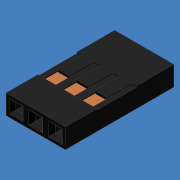
# Autodesk Inventor part: PMW_Terminal
Saved by Autodesk Inventor 2012 (Build 160160000, 160)
## iProperties
Company: Team 801
Created: 2006-06-02
Part Number: PMW_Terminal
Document SubType Name: Modeling
Designer: Jeffrey M
Catalog Web Link: www.team801.org
Density: 1 g/cm^3
Material: Default
Author: Jeffrey M
Autodesk Inventor part; units mm, degrees
ref_plane "YZ Plane" through (0, 0, 0) normal (1, 0, 0) x (0, 1, 0)
ref_plane "XZ Plane" through (0, 0, 0) normal (0, 1, 0) x (-1, 0, 0)
ref_plane "XY Plane" through (0, 0, 0) normal (0, 0, 1) x (1, 0, 0)
sketch "Sketch1" plane through (0, 0, 0) normal (0, 0, 1) x (1, 0, 0)
  line L0 (-23.5871, -5.7068) -> (-15.9671, -5.7068)
  line L1 (-15.9671, -5.7068) -> (-15.9671, -8.2468)
  line L2 (-15.9671, -8.2468) -> (-23.5871, -8.2468)
  line L3 (-23.5871, -8.2468) -> (-23.5871, -5.7068)
  dimension "d0" = 2.54
  dimension "d1" = 7.62
  constraints: 8 end point, 2 parallel, 1 horizontal, 1 perpendicular
  measures "d0" distance of L2.end L0.start
  measures "d1" distance of L0.start L0.end
extrude "Extrusion1" add sketch "Sketch1" along normal blind 13.97
sketch "Sketch2" plane through (0, 0, 13.97) normal (0, 0, 1) x (1, 0, 0)
  line L0 (-23.5871, -5.7068) -> (-15.9671, -5.7068) projected
  line L1 (-23.5871, -8.2468) -> (-23.5871, -5.7068) projected
  line L2 (-15.9671, -8.2468) -> (-23.5871, -8.2468) projected
  line L3 (-23.2061, -6.0878) -> (-21.4281, -6.0878)
  line L4 (-21.4281, -6.0878) -> (-21.4281, -7.8658)
  line L5 (-21.4281, -7.8658) -> (-23.2061, -7.8658)
  line L6 (-23.2061, -7.8658) -> (-23.2061, -6.0878)
  line L7 (-19.7771, -5.7068) -> (-19.7771, -5.9181)
  line L8 (-16.3481, -6.0878) -> (-18.1261, -6.0878)
  line L9 (-18.1261, -6.0878) -> (-18.1261, -7.8658)
  line L10 (-18.1261, -7.8658) -> (-16.3481, -7.8658)
  line L11 (-16.3481, -7.8658) -> (-16.3481, -6.0878)
  line L12 (-20.6661, -6.0878) -> (-18.8881, -6.0878)
  line L13 (-18.8881, -6.0878) -> (-18.8881, -7.8658)
  line L14 (-18.8881, -7.8658) -> (-20.6661, -7.8658)
  line L15 (-20.6661, -7.8658) -> (-20.6661, -6.0878)
  dimension "d4" = 0.381
  dimension "d5" = 0.381
  dimension "d6" = 0.381
  dimension "d7" = 1.778
  dimension "d8" = 1.778
  dimension "d9" = 1.778
  dimension "d10" = 0.762
  dimension "d11" = 0.762
  constraints: 26 end point, 5 parallel, 4 symmetric about line, 2 horizontal, 2 perpendicular, 1 midpoint
  measures "d4" distance between parallel lines of L1 L6
  measures "d5" distance between parallel lines of L0 L3
  measures "d6" distance between parallel lines of L2 L5
  measures "d7" distance of L3.start L3.end
  measures "d8" distance of L12.start L12.end
  measures "d9" distance of L12.end L13.end
  measures "d10" distance between parallel lines of L15 L4
  measures "d11" distance between parallel lines of L9 L13
extrude "Extrusion2" cut sketch "Sketch2" against normal blind 0.381 draft -50
sketch "Sketch3" plane through (0, 0, 13.589) normal (0, 0, 1) x (1, 0, 0)
  line L0 (-22.752, -6.5419) -> (-22.752, -7.4118) projected
  line L1 (-22.752, -7.4118) -> (-21.8821, -7.4118) projected
  line L2 (-21.8821, -7.4118) -> (-21.8821, -6.5419) projected
  line L3 (-21.8821, -6.5419) -> (-22.752, -6.5419) projected
  line L4 (-20.212, -6.5419) -> (-20.212, -7.4118) projected
  line L5 (-20.212, -7.4118) -> (-19.3421, -7.4118) projected
  line L6 (-19.3421, -7.4118) -> (-19.3421, -6.5419) projected
  line L7 (-19.3421, -6.5419) -> (-20.212, -6.5419) projected
  line L8 (-17.672, -6.5419) -> (-17.672, -7.4118) projected
  line L9 (-17.672, -7.4118) -> (-16.8021, -7.4118) projected
  line L10 (-16.8021, -7.4118) -> (-16.8021, -6.5419) projected
  line L11 (-16.8021, -6.5419) -> (-17.672, -6.5419) projected
extrude "Extrusion3" cut sketch "Sketch3" against normal through all
sketch "Sketch4" plane through (0, 0, 0) normal (0, 0, -1) x (-1, 0, 0)
  line L0 (20.212, -7.4118) -> (19.3421, -7.4118) projected
  line L1 (19.3421, -7.4118) -> (19.3421, -6.5419) projected
  line L2 (19.3421, -6.5419) -> (20.212, -6.5419) projected
  line L3 (20.212, -6.5419) -> (20.212, -7.4118) projected
  line L4 (22.752, -7.4118) -> (21.8821, -7.4118) projected
  line L5 (21.8821, -7.4118) -> (21.8821, -6.5419) projected
  line L6 (21.8821, -6.5419) -> (22.752, -6.5419) projected
  line L7 (22.752, -6.5419) -> (22.752, -7.4118) projected
  line L8 (17.672, -7.4118) -> (16.8021, -7.4118) projected
  line L9 (16.8021, -7.4118) -> (16.8021, -6.5419) projected
  line L10 (16.8021, -6.5419) -> (17.672, -6.5419) projected
  line L11 (17.672, -6.5419) -> (17.672, -7.4118) projected
  line L12 (23.2696, -6.0243) -> (21.3646, -6.0243)
  line L13 (21.3646, -6.0243) -> (21.3646, -7.9293)
  line L14 (21.3646, -7.9293) -> (23.2696, -7.9293)
  line L15 (23.2696, -7.9293) -> (23.2696, -6.0243)
  line L16 (18.1896, -6.0243) -> (16.2846, -6.0243)
  line L17 (16.2846, -6.0243) -> (16.2846, -7.9293)
  line L18 (16.2846, -7.9293) -> (18.1896, -7.9293)
  line L19 (18.1896, -7.9293) -> (18.1896, -6.0243)
  line L20 (20.7296, -6.0243) -> (18.8246, -6.0243)
  line L21 (18.8246, -6.0243) -> (18.8246, -7.9293)
  line L22 (18.8246, -7.9293) -> (20.7296, -7.9293)
  line L23 (20.7296, -7.9293) -> (20.7296, -6.0243)
  dimension "d16" = 1.905
  constraints: 24 end point, 2 collinear, 9 other
  measures "d16" distance of L14.end L12.start
extrude "Extrusion4" cut sketch "Sketch4" against normal blind 3.175
sketch "Sketch5" plane through (-23.5871, -5.7068, 0) normal (0, 1, 0) x (1, 0, 0)
  line L0 (7.62, 0) -> (7.62, -13.97) projected
  line L1 (0, 0) -> (0, -13.97) projected
  line L2 (0, -4.826) -> (7.62, -4.826)
  line L3 (7.62, -4.826) -> (7.62, -9.906)
  line L4 (7.62, -9.906) -> (0, -9.906)
  line L5 (0, -9.906) -> (0, -4.826)
  line L6 (0.635, -9.906) -> (2.159, -9.906)
  line L7 (2.159, -9.906) -> (2.159, -8.001)
  line L8 (2.159, -8.001) -> (0.635, -8.001)
  line L9 (0.635, -8.001) -> (0.635, -9.906)
  line L10 (3.81, -9.906) -> (5.334, -9.906)
  line L11 (5.461, -9.906) -> (6.985, -9.906)
  line L12 (6.985, -9.906) -> (6.985, -8.001)
  line L13 (6.985, -8.001) -> (5.461, -8.001)
  line L14 (5.461, -8.001) -> (5.461, -9.906)
  line L15 (3.048, -9.906) -> (4.572, -9.906)
  line L16 (4.572, -9.906) -> (4.572, -8.001)
  line L17 (4.572, -8.001) -> (3.048, -8.001)
  line L18 (3.048, -8.001) -> (3.048, -9.906)
  line L19 (0.635, -8.001) -> (2.159, -8.001)
  line L20 (2.159, -8.001) -> (2.159, -4.826)
  line L21 (2.159, -4.826) -> (0.635, -4.826)
  line L22 (0.635, -4.826) -> (0.635, -8.001)
  line L23 (3.048, -8.001) -> (4.572, -8.001)
  line L24 (4.572, -8.001) -> (4.572, -4.826)
  line L25 (4.572, -4.826) -> (3.048, -4.826)
  line L26 (3.048, -4.826) -> (3.048, -8.001)
  line L27 (5.461, -8.001) -> (6.985, -8.001)
  line L28 (6.985, -8.001) -> (6.985, -4.826)
  line L29 (6.985, -4.826) -> (5.461, -4.826)
  line L30 (5.461, -4.826) -> (5.461, -8.001)
  line L31 (0, -13.97) -> (7.62, -13.97) projected
  line L32 (0.635, -8.001) -> (2.159, -8.001)
  line L33 (2.159, -8.001) -> (2.159, -9.906)
  line L34 (2.159, -9.906) -> (0.635, -9.906)
  line L35 (0.635, -9.906) -> (0.635, -8.001)
  dimension "d19" = 5.08
  dimension "d21" = 1.524
  dimension "d23" = 0.889
  dimension "d24" = 0.889
  dimension "d25" = 0.635
  dimension "d30" = 3.175
  dimension "d31" = 4.064
  constraints: 66 end point, 19 equal length, 8 perpendicular, 7 collinear, 6 horizontal, 6 point on line, 1 midpoint
  measures "d19" distance of L2.end L3.end
  measures "d21" distance of L7.end L8.end
  measures "d23" distance between parallel lines of L7 L18
  measures "d24" distance between parallel lines of L14 L16
  measures "d25" distance between parallel lines of L1 L9
  measures "d30" distance between parallel lines of L2 L13
  measures "d31" distance between parallel lines of L31 L4
extrude "Extrusion6" cut sketch "Sketch5" against normal blind 0.3175 contours L4 L14 L13 L12 | L16 L4 L18 L17 | L9 L8 L7 L4
extrude "Extrusion7" cut sketch "Sketch5" against normal blind 0.1588 contours L0 L4 L12 L28 L2 | L30 L14 L4 L16 L24 L2 | L1 L2 L22 L9 L4 | L26 L18 L4 L7 L20 L2
sketch "Sketch6" plane through (0, 0, 3.175) normal (0, 0, -1) x (-1, 0, 0)
  line L0 (17.672, -7.4118) -> (17.672, -6.5419) projected
  line L1 (16.8021, -7.4118) -> (17.672, -7.4118) projected
  line L2 (16.8021, -6.5419) -> (16.8021, -7.4118) projected
  line L3 (17.672, -6.5419) -> (16.8021, -6.5419) projected
  line L4 (16.2846, -6.0243) -> (16.2846, -7.9293) projected
  line L5 (16.2846, -7.9293) -> (18.1896, -7.9293) projected
  line L6 (18.1896, -7.9293) -> (18.1896, -6.0243) projected
  line L7 (18.1896, -6.0243) -> (16.2846, -6.0243) projected
  line L8 (20.212, -7.4118) -> (20.212, -6.5419) projected
  line L9 (19.3421, -7.4118) -> (20.212, -7.4118) projected
  line L10 (19.3421, -6.5419) -> (19.3421, -7.4118) projected
  line L11 (20.212, -6.5419) -> (19.3421, -6.5419) projected
  line L12 (18.8246, -6.0243) -> (18.8246, -7.9293) projected
  line L13 (18.8246, -7.9293) -> (20.7296, -7.9293) projected
  line L14 (20.7296, -7.9293) -> (20.7296, -6.0243) projected
  line L15 (20.7296, -6.0243) -> (18.8246, -6.0243) projected
  line L16 (22.752, -7.4118) -> (22.752, -6.5419) projected
  line L17 (21.8821, -7.4118) -> (22.752, -7.4118) projected
  line L18 (21.8821, -6.5419) -> (21.8821, -7.4118) projected
  line L19 (22.752, -6.5419) -> (21.8821, -6.5419) projected
  line L20 (21.3646, -6.0243) -> (21.3646, -7.9293) projected
  line L21 (21.3646, -7.9293) -> (23.2696, -7.9293) projected
  line L22 (23.2696, -7.9293) -> (23.2696, -6.0243) projected
  line L23 (23.2696, -6.0243) -> (21.3646, -6.0243) projected
  point P0 (17.2371, -6.9768)
  point P1 (19.7771, -6.9768)
  point P2 (22.3171, -6.9768)
body "Solid1"
